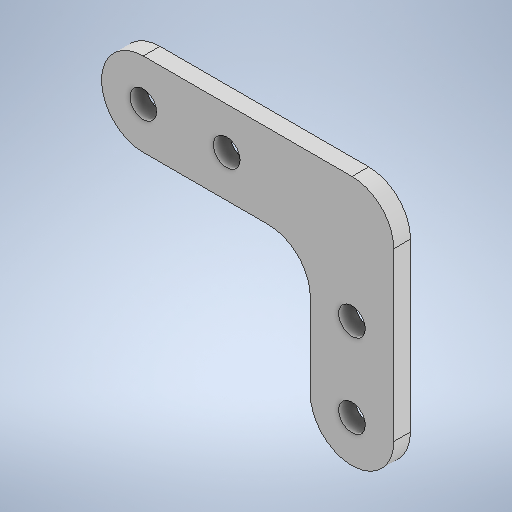
# Autodesk Inventor part: kakutome_nc
Saved by Autodesk Inventor 2025.1 (Build 291241000, 241)
## iProperties
Created: 2025-05-05
Part Number: kakutome_nc
Material: 一般
Document SubType Name: Modeling
Designer: yuki0520
Density: 1 g/cm^3
Appearance: 既定
Author: yuki0520
Autodesk Inventor part; units mm, degrees
ref_plane "YZ Plane" through (0, 0, 0) normal (1, 0, 0) x (0, 1, 0)
ref_plane "XZ Plane" through (0, 0, 0) normal (0, 1, 0) x (-1, 0, 0)
ref_plane "XY Plane" through (0, 0, 0) normal (0, 0, 1) x (1, 0, 0)
sketch "スケッチ1" plane through (0, 0, 0) normal (0, 0, 1) x (1, 0, 0)
  line L0 (0, 0) -> (-10, 0)
  line L1 (-10, 0) -> (-10, -20)
  line L2 (-10, -20) -> (0, -20)
  line L3 (0, -20) -> (0, 0)
  line L4 (0, 0) -> (-35, 0)
  line L5 (-35, 0) -> (-35, 10)
  line L6 (-35, 10) -> (0, 10)
  line L7 (0, 10) -> (0, 0)
  line L8 (-5, -20) -> (-5, 0)
  line L9 (0, 5) -> (-35, 5)
  circle A0 centre (-10, 5) radius 1.6
  circle A1 centre (-5, -5) radius 1.6
  circle A2 centre (-20, 5) radius 1.6
  circle A3 centre (-30, 5) radius 1.6
  circle A4 centre (-5, -15) radius 1.6
  circle A5 centre (-5, -25) radius 1.6
  dimension "d0" = 10
  dimension "d1" = 20
  dimension "d2" = 35
  dimension "d3" = 10
  dimension "d4" = 3.2
  dimension "d5" = 3.2
  dimension "d6" = 10
  dimension "d7" = 5
  dimension "d11" = 10
  dimension "d18" = 10
  constraints: 20 end point, 6 centre point, 4 parallel, 3 horizontal, 3 midpoint, 3 perpendicular, 3 point on line, 1 vertical, 8 other
  measures "d0" distance of L2.end L1.end
  measures "d1" distance of L1.end L0.end
  measures "d2" distance of L5.end L6.end
  measures "d3" distance of L4.end L5.end
  measures "d4" diameter of A0
  measures "d5" diameter of A1
  measures "d6" distance from line of L7 A0.centre
  measures "d7" distance from line of L0 A1.centre
  measures "d11" distance of A0.centre A2.centre
  measures "d18" distance of A1.centre A4.centre
extrude "押し出し1" add sketch "スケッチ1" along normal blind 2 contours L3 L2 L8 A4 A1 L0 | L0 L4 L5 L9 A3 A2 A0 L7 | L8 A1 A4 L2 L1 L0 | L9 A0 A2 A3 L5 L6 L7 | A0 L9 | L9 A0
fillet "フィレット1" radius 5 6 edges at (0, 10, 1) (-35, 10, 1) (-35, 0, 1) (0, -20, 1) (-10, -20, 1) (-10, 0, 1)
